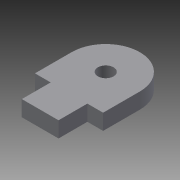
# Autodesk Inventor part: Gripper V 6.0 base tab 3mm
Saved by Autodesk Inventor 2015 (Build 190159000, 159)
## iProperties
Created: 2015-06-11
Part Number: Gripper V 6.0 base tab 3mm
Material: Generic
Document SubType Name: Modeling
Designer: Stackpole
Density: 1 g/cm^3
Appearance: Default
Author: Stackpole
Autodesk Inventor part; units mm, degrees
ref_plane "YZ Plane" through (0, 0, 0) normal (1, 0, 0) x (0, 1, 0)
ref_plane "XZ Plane" through (0, 0, 0) normal (0, 1, 0) x (-1, 0, 0)
ref_plane "XY Plane" through (0, 0, 0) normal (0, 0, 1) x (1, 0, 0)
sketch "Sketch1" plane through (0, 0, 0) normal (0, 0, 1) x (1, 0, 0)
  line L0 (13, 0) -> (13, 7)
  line L1 (0, 7) -> (0, 0)
  arc A0 (13, 7) -> (0, 7) centre (6.5, 7) ccw
  line L2 (10, 0) -> (10, -5.5)
  line L3 (10, -5.5) -> (3, -5.5)
  line L4 (3, -5.5) -> (3, 0)
  line L5 (0, 0) -> (3, 0)
  line L6 (10, 0) -> (13, 0)
  circle A1 centre (6.5, 7) radius 1.5
  dimension "d0" = 7
  dimension "d1" = 3
  dimension "d2" = 3
  dimension "d3" = 7
  dimension "d7" = 3
  dimension "d10" = 5.5
  dimension "d11" = 7
  constraints: 14 end point, 2 centre point, 2 horizontal, 2 parallel, 2 perpendicular, 2 point on circle, 2 tangent, 1 coincident
  measures "d0" distance of L2.end L3.end
  measures "d1" distance of L2.start L0.start
  measures "d2" distance of L1.end L4.end
  measures "d3" distance of L0.start L0.end
  measures "d7" diameter of A1
  measures "d10" distance between parallel lines of L3 L6
  measures "d11" distance of L1.start L1.end
extrude "Extrusion2" add sketch "Sketch1" along normal blind 3
body "Solid2"
